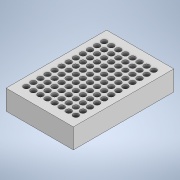
# Autodesk Inventor part: PTFE casting tray
Saved by Autodesk Inventor 2020 (Build 240168000, 168)
## iProperties
Created: 2021-10-05
Part Number: PTFE casting tray
Material: Generic
Document SubType Name: Modeling
Designer: pab2
Density: 1 g/cm^3
Appearance: Default
Author: pab2
Autodesk Inventor part; units mm, degrees
ref_plane "YZ Plane" through (0, 0, 0) normal (1, 0, 0) x (0, 1, 0)
ref_plane "XZ Plane" through (0, 0, 0) normal (0, 1, 0) x (-1, 0, 0)
ref_plane "XY Plane" through (0, 0, 0) normal (0, 0, 1) x (1, 0, 0)
sketch "Sketch1" plane through (0, 0, 0) normal (0, 1, 0) x (-1, 0, 0)
  line L0 (0, 0) -> (-85.471, 0)
  line L1 (-85.471, 0) -> (-85.471, 127.762)
  line L2 (-85.471, 127.762) -> (0, 127.762)
  line L3 (0, 127.762) -> (0, 0)
  dimension "d0" = 85.471
  dimension "d1" = 127.762
  constraints: 8 end point, 2 parallel, 1 horizontal, 1 perpendicular
  measures "d0" distance of L1.end L2.end
  measures "d1" distance of L0.end L1.end
extrude "Extrusion1" add sketch "Sketch1" along normal blind 25.4
sketch "Sketch2" plane through (0, 25.4, 0) normal (0, 1, 0) x (1, 0, 0)
  line L0 (85.471, 0) -> (0, 0) projected
  line L1 (0, 0) -> (11.2395, 0)
  line L2 (11.2395, 0) -> (11.2395, -14.3789)
  line L3 (11.2395, -14.3789) -> (0, -14.3789)
  line L4 (0, -14.3789) -> (0, 0)
  circle A0 centre (11.2395, -14.3789) radius 3.5
  dimension "d4" = 11.2395
  dimension "d5" = 14.3789
  dimension "d6" = 7
  constraints: 8 end point, 2 parallel, 1 centre point, 1 coincident, 1 horizontal, 1 perpendicular
  measures "d4" distance of L2.end L3.end
  measures "d5" distance of L1.end L2.end
  measures "d6" diameter of A0
hole "Hole1" at (11.2395, 25.4, 14.3789) direction (0, -1, 0) diameter 7 end through all
pattern_linear "Rectangular Pattern1" count 8 spacing 9 along (1, 0, 0) count 12 spacing 9 along (0, 0, 1) of "Hole1"
body "Solid1"
